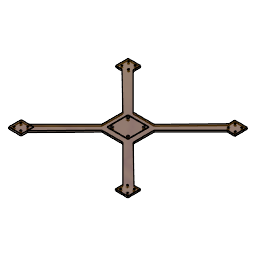
quadcopter_frame_v3 (Autodesk Fusion 360 design; units mm, degrees)
part number: 2025-07-17-20-15-15-900
Autodesk Fusion 360 part; units mm, degrees
note: some values were not read from the file. Set by a fixed rule: which sketch regions a step uses.
sketch "Sketch1" plane through (0, 0, 0) normal (0, 0, 1) x (1, 0, 0)
  line L0 (19.9391, 19.9391) -> (-19.9391, 19.9391)
  line L1 (-19.9391, 19.9391) -> (-19.9391, -19.9391)
  line L2 (-19.9391, -19.9391) -> (19.9391, -19.9391)
  line L3 (19.9391, -19.9391) -> (19.9391, 19.9391)
  line L4 (19.9391, 19.9391) -> (-19.9391, -19.9391) construction
  line L5 (-19.9391, 19.9391) -> (19.9391, -19.9391) construction
  line L6 (30, 30) -> (-30, 30)
  line L7 (-30, 30) -> (-30, -30)
  line L8 (-30, -30) -> (30, -30)
  line L9 (30, -30) -> (30, 30)
  line L10 (30, 30) -> (-30, -30) construction
  line L11 (-30, 30) -> (30, -30) construction
  circle A0 centre (-15.25, 15.25) radius 2
  circle A1 centre (15.2506, 15.2506) radius 2
  circle A2 centre (15.2785, -15.2785) radius 2
  circle A3 centre (-15.2506, -15.2506) radius 2
  line L12 (-20, -30) -> (105, -30) construction
  line L13 (-30, -20) -> (95, -20) construction
  line L14 (-30, 20) -> (95, 20) construction
  line L15 (30, 20) -> (155, 20) construction
  line L16 (-20, -30) -> (-90.3727, -102)
  line L17 (-30, -20) -> (-100, -90)
  line L18 (-90.3727, -90) -> (-114.3727, -90)
  line L19 (-90.3727, -90) -> (-90.3727, -114)
  line L20 (-114.3727, -114) -> (-114.3727, -90)
  line L21 (-90.3727, -114) -> (-114.3727, -114)
  circle A4 centre (-109.5, -108.5) radius 1.5
  circle A5 centre (-96.5, -108.5) radius 1.5
  circle A6 centre (-96.5, -95.5) radius 1.5
  circle A7 centre (-109.5, -95.5) radius 1.5
  line L22 (30, -20) -> (102, -90.3727)
  line L23 (20, -30) -> (90, -100)
  line L24 (20, 30) -> (90.3727, 102)
  line L25 (30, 20) -> (100, 90)
  line L26 (-30, 20) -> (-102, 90.3727)
  line L27 (-20, 30) -> (-90, 100)
  circle A8 centre (95.5, -109.5) radius 1.5
  circle A9 centre (95.5, -96.5) radius 1.5
  circle A10 centre (108.5, -109.5) radius 1.5
  circle A11 centre (108.5, -96.5) radius 1.5
  line L28 (114, -90.3727) -> (114, -114.3727)
  line L29 (90, -90.3727) -> (114, -90.3727)
  line L30 (90, -90.3727) -> (90, -114.3727)
  line L31 (114, -114.3727) -> (90, -114.3727)
  circle A12 centre (109.5, 95.5) radius 1.5
  circle A13 centre (96.5, 95.5) radius 1.5
  circle A14 centre (109.5, 108.5) radius 1.5
  circle A15 centre (96.5, 108.5) radius 1.5
  line L32 (90.3727, 114) -> (114.3727, 114)
  line L33 (90.3727, 90) -> (90.3727, 114)
  line L34 (90.3727, 90) -> (114.3727, 90)
  line L35 (114.3727, 114) -> (114.3727, 90)
  circle A16 centre (-95.5, 109.5) radius 1.5
  circle A17 centre (-95.5, 96.5) radius 1.5
  circle A18 centre (-108.5, 109.5) radius 1.5
  circle A19 centre (-108.5, 96.5) radius 1.5
  line L36 (-114, 90.3727) -> (-114, 114.3727)
  line L37 (-90, 90.3727) -> (-114, 90.3727)
  line L38 (-90, 90.3727) -> (-90, 114.3727)
  line L39 (-114, 114.3727) -> (-90, 114.3727)
  dimension "d69" = 360
  constraint horizontal L0
  constraint perpendicular L0 L1
  constraint parallel L0 L2
  constraint parallel L1 L3
  constraint coincident L4 origin
  constraint coincident L5 origin
  constraint horizontal L6
  constraint perpendicular L6 L7
  constraint parallel L6 L8
  constraint parallel L7 L9
  constraint coincident L10 origin
  constraint coincident L11 origin
  constraint coincident L11 A0.centre
  constraint coincident L4 A1.centre
  constraint coincident L5 A2.centre
  constraint coincident L4 A3.centre
  constraint horizontal L12
  constraint coincident L8 L12.start
  constraint horizontal L13
  constraint coincident L7 L13.start
  constraint horizontal L14
  constraint coincident L7 L14.start
  constraint horizontal L15
  constraint coincident L14 L15.start
  constraint coincident L9 L15.start
extrude "Extrude10" add sketch "Sketch1" along normal blind 3 contours L6 L7 L8 L9 | L6 L9 L24 L25 L33 L34 | L6 L7 L26 L27 L37 L38 | L8 L9 L22 L23 L29 L30 | L7 L8 L16 L17 L18 L19
extrude "Extrude11" add sketch "Sketch1" along normal blind 3.5 contours L18 L19 L20 L21
extrude "Extrude12" add sketch "Sketch1" along normal blind 3.5 contours L0 L1 L2 L3
extrude "Extrude13" add sketch "Sketch1" along normal blind 3 contours L32 L33 L34 L35 | L36 L37 L38 L39 | L28 L29 L30 L31
sketch "Sketch2" plane through (0, 0, 0) normal (0, 0, 1) x (1, 0, 0)
extrude "Extrude6" [suppressed]
extrude "Extrude7" [suppressed]
extrude "Extrude8" [suppressed]
extrude "Extrude9" [suppressed]
